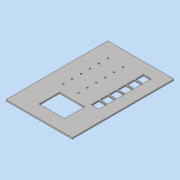
# Autodesk Inventor part: panel
Saved by Autodesk Inventor 2016 (Build 200138000, 138)
## iProperties
Created: 2016-07-20
Part Number: panel
Material: Generic
Document SubType Name: Modeling
Designer: Zuhra Abdurashidova
Density: 1 g/cm^3
Appearance: Default
Author: Zuhra Abdurashidova
Autodesk Inventor part; units mm, degrees
ref_plane "YZ Plane" through (0, 0, 0) normal (1, 0, 0) x (0, 1, 0)
ref_plane "XZ Plane" through (0, 0, 0) normal (0, 1, 0) x (-1, 0, 0)
ref_plane "XY Plane" through (0, 0, 0) normal (0, 0, 1) x (1, 0, 0)
sketch "Sketch1" plane through (0, 0, 0) normal (0, 1, 0) x (-1, 0, 0)
  line L0 (0, 0) -> (-330.2, 0)
  line L1 (-330.2, 0) -> (-330.2, -508)
  line L2 (-330.2, -508) -> (0, -508)
  line L3 (0, -508) -> (0, 0)
  line L4 (-73.0377, -433.3) -> (-73.0377, -430.3)
  arc A0 (-73.0377, -430.3) -> (-73.0377, -433.3) centre (-76.2, -431.8) ccw
  line L5 (-149.2377, -433.3) -> (-149.2377, -430.3)
  arc A1 (-149.2377, -430.3) -> (-149.2377, -433.3) centre (-152.4, -431.8) ccw
  line L6 (-73.0377, -388.85) -> (-73.0377, -385.85)
  arc A2 (-73.0377, -385.85) -> (-73.0377, -388.85) centre (-76.2, -387.35) ccw
  line L7 (-149.2377, -388.85) -> (-149.2377, -385.85)
  arc A3 (-149.2377, -385.85) -> (-149.2377, -388.85) centre (-152.4, -387.35) ccw
  line L8 (-73.0377, -344.4) -> (-73.0377, -341.4)
  arc A4 (-73.0377, -341.4) -> (-73.0377, -344.4) centre (-76.2, -342.9) ccw
  line L9 (-149.2377, -344.4) -> (-149.2377, -341.4)
  arc A5 (-149.2377, -341.4) -> (-149.2377, -344.4) centre (-152.4, -342.9) ccw
  line L10 (-73.0377, -299.95) -> (-73.0377, -296.95)
  arc A6 (-73.0377, -296.95) -> (-73.0377, -299.95) centre (-76.2, -298.45) ccw
  line L11 (-149.2377, -299.95) -> (-149.2377, -296.95)
  arc A7 (-149.2377, -296.95) -> (-149.2377, -299.95) centre (-152.4, -298.45) ccw
  line L12 (-73.0377, -255.5) -> (-73.0377, -252.5)
  arc A8 (-73.0377, -252.5) -> (-73.0377, -255.5) centre (-76.2, -254) ccw
  line L13 (-149.2377, -255.5) -> (-149.2377, -252.5)
  arc A9 (-149.2377, -252.5) -> (-149.2377, -255.5) centre (-152.4, -254) ccw
  line L14 (-73.0377, -211.05) -> (-73.0377, -208.05)
  arc A10 (-73.0377, -208.05) -> (-73.0377, -211.05) centre (-76.2, -209.55) ccw
  line L15 (-149.2377, -211.05) -> (-149.2377, -208.05)
  arc A11 (-149.2377, -208.05) -> (-149.2377, -211.05) centre (-152.4, -209.55) ccw
  line L16 (-234.95, -412.75) -> (-273.05, -412.75)
  line L17 (-273.05, -412.75) -> (-273.05, -450.85)
  line L18 (-273.05, -450.85) -> (-234.95, -450.85)
  line L19 (-234.95, -450.85) -> (-234.95, -412.75)
  line L20 (-234.95, -412.75) -> (-273.05, -450.85) construction
  line L21 (-273.05, -412.75) -> (-234.95, -450.85) construction
  line L22 (-234.95, -368.3) -> (-273.05, -368.3)
  line L23 (-234.95, -406.4) -> (-234.95, -368.3)
  line L24 (-273.05, -368.3) -> (-273.05, -406.4)
  line L25 (-273.05, -406.4) -> (-234.95, -406.4)
  line L26 (-273.05, -368.3) -> (-234.95, -406.4) construction
  line L27 (-234.95, -368.3) -> (-273.05, -406.4) construction
  line L28 (-234.95, -323.85) -> (-273.05, -323.85)
  line L29 (-234.95, -361.95) -> (-234.95, -323.85)
  line L30 (-273.05, -323.85) -> (-273.05, -361.95)
  line L31 (-273.05, -361.95) -> (-234.95, -361.95)
  line L32 (-273.05, -323.85) -> (-234.95, -361.95) construction
  line L33 (-234.95, -323.85) -> (-273.05, -361.95) construction
  line L34 (-234.95, -279.4) -> (-273.05, -279.4)
  line L35 (-234.95, -317.5) -> (-234.95, -279.4)
  line L36 (-273.05, -279.4) -> (-273.05, -317.5)
  line L37 (-273.05, -317.5) -> (-234.95, -317.5)
  line L38 (-273.05, -279.4) -> (-234.95, -317.5) construction
  line L39 (-234.95, -279.4) -> (-273.05, -317.5) construction
  line L40 (-234.95, -234.95) -> (-273.05, -234.95)
  line L41 (-234.95, -273.05) -> (-234.95, -234.95)
  line L42 (-273.05, -234.95) -> (-273.05, -273.05)
  line L43 (-273.05, -273.05) -> (-234.95, -273.05)
  line L44 (-273.05, -234.95) -> (-234.95, -273.05) construction
  line L45 (-234.95, -234.95) -> (-273.05, -273.05) construction
  line L46 (-234.95, -190.5) -> (-273.05, -190.5)
  line L47 (-234.95, -228.6) -> (-234.95, -190.5)
  line L48 (-273.05, -190.5) -> (-273.05, -228.6)
  line L49 (-273.05, -228.6) -> (-234.95, -228.6)
  line L50 (-273.05, -190.5) -> (-234.95, -228.6) construction
  line L51 (-234.95, -190.5) -> (-273.05, -228.6) construction
  line L52 (-101.6, -165.1) -> (-228.6, -165.1)
  line L53 (-228.6, -165.1) -> (-228.6, -63.5)
  line L54 (-228.6, -63.5) -> (-101.6, -63.5)
  line L55 (-101.6, -63.5) -> (-101.6, -165.1)
  point P0 (-254, -431.8)
  point P1 (-254, -387.35)
  point P2 (-254, -342.9)
  point P3 (-254, -298.45)
  point P4 (-254, -254)
  point P5 (-254, -209.55)
  dimension "d0" = 330.2
  dimension "d1" = 508
  dimension "d107" = 3.5
  dimension "d109" = 3
  dimension "d111" = 76.2
  dimension "d135" = 76.2
  dimension "d138" = 76.2
  dimension "d141" = 44.45
  dimension "d144" = 38.1
  dimension "d145" = 38.1
  dimension "d146" = 76.2
  dimension "d147" = 76.2
  dimension "d150" = 44.45
  dimension "d155" = 101.6
  dimension "d156" = 127
  dimension "d157" = 101.6
  dimension "d158" = 63.5
  constraints: 112 end point, 24 point on circle, 12 centre point, 12 midpoint, 6 parallel, 4 horizontal, 3 perpendicular, 3 vertical, 110 other
  measures "d0" distance of L1.end L2.end
  measures "d1" distance of L0.end L1.end
  measures "d107" radius of A0
  measures "d109" distance of L4.start L4.end
  measures "d111" distance from line of L2 A0.centre
  measures "d135" distance from line of A0.centre L3
  measures "d138" distance of L4.start L5.start
  measures "d141" distance of L4.start L6.start
  measures "d144" distance of L17.end L18.end
  measures "d145" distance of L16.end L17.end
  measures "d146" distance from line of L2 point (-254, -431.8)
  measures "d147" distance from line of L1 point (-254, -431.8)
  measures "d150" distance of L16.start L22.start
  measures "d155" distance of L52.end L53.end
  measures "d156" distance of L52.start L52.end
  measures "d157" distance between parallel lines of L53 L1
  measures "d158" distance between parallel lines of L54 L0
extrude "panel body" add sketch "Sketch1" along normal blind 6.35
body "Solid3"
